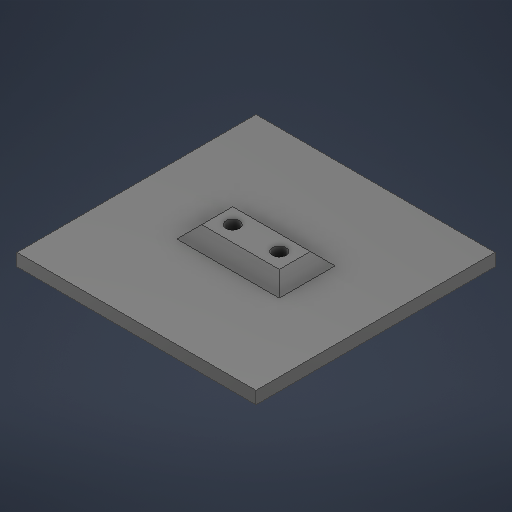
# Autodesk Inventor part: taca
Saved by Autodesk Inventor 2027 (Build 310192060, 192F)
## iProperties
Created: 2026-03-26
Part Number: taca
Material: Ogólny
Document SubType Name: Modeling
Designer: User
Density: 1 g/cm^3
Appearance: Domyślna
Author: User
Autodesk Inventor part; units mm, degrees
ref_plane "YZ Plane" through (0, 0, 0) normal (1, 0, 0) x (0, 1, 0)
ref_plane "XZ Plane" through (0, 0, 0) normal (0, 1, 0) x (-1, 0, 0)
ref_plane "XY Plane" through (0, 0, 0) normal (0, 0, 1) x (1, 0, 0)
sketch "Szkic1" plane through (0, 0, 0) normal (0, 1, 0) x (-1, 0, 0)
  line L0 (0, 0) -> (7.5, 0)
  line L1 (0, 0) -> (7.5, 0) construction
  circle A0 centre (7.5, 0) radius 2.2
  line L2 (0, 0) -> (0, -2)
  circle A1 centre (-7.5, 0) radius 2.2
  line L3 (-38.5, 38.5) -> (38.5, 38.5)
  line L4 (38.5, 38.5) -> (38.5, -38.5)
  line L5 (38.5, -38.5) -> (-38.5, -38.5)
  line L6 (-38.5, -38.5) -> (-38.5, 38.5)
  line L7 (-38.5, 38.5) -> (38.5, -38.5) construction
  line L8 (38.5, 38.5) -> (-38.5, -38.5) construction
  circle A2 centre (7.5, 0) radius 3.5
  circle A3 centre (-7.5, 0) radius 3.5
  dimension "d0" = 7.5
  dimension "d1" = 0
  dimension "d2" = 4.4
  dimension "d3" = 2
  dimension "d4" = 77
  dimension "d5" = 77
  dimension "d8" = 7
  constraints: 18 end point, 4 centre point, 3 horizontal, 2 coincident, 2 midpoint, 2 parallel, 2 symmetric about line, 1 collinear, 1 perpendicular, 1 vertical, 2 other
  measures "d0" distance of L0.start L0.end
  measures "d1" distance between parallel lines of L0 L1
  measures "d2" diameter of A0
  measures "d3" distance of L0.start L2.end
  measures "d4" distance of L4.end L5.end
  measures "d5" distance of L3.end L4.end
  measures "d8" diameter of A2
extrude "Wyciągnięcie proste1" add sketch "Szkic1" along normal blind 6 contours A2 | L3 L4 L5 L6 | A3
extrude "Wyciągnięcie proste2" cut sketch "Szkic1" along normal blind 3 contours A2 | A3
chamfer "Faza1" distance 2 angle 45 4 edges at (-38.5, 0, 0) (0, 0, -38.5) (38.5, 0, 0) (0, 0, 38.5)
sketch "Szkic2" plane through (0, 6, 0) normal (0, 1, 0) x (1, 0, 0)
  line L0 (12.5, -5) -> (-12.5, -5)
  line L1 (-12.5, -5) -> (-12.5, 5)
  line L2 (-12.5, 5) -> (12.5, 5)
  line L3 (12.5, 5) -> (12.5, -5)
  line L4 (12.5, -5) -> (-12.5, 5) construction
  line L5 (-12.5, -5) -> (12.5, 5) construction
  circle A0 centre (-7.5, 0) radius 2.2 projected
  circle A1 centre (-7.5, 0) radius 2.2
  circle A2 centre (7.5, 0) radius 2.2 projected
  circle A3 centre (7.5, 0) radius 2.2
  point P0 (0, 0)
  dimension "d14" = 25
  dimension "d15" = 10
  constraints: 12 end point, 2 centre point, 2 coincident, 2 midpoint, 2 parallel, 1 horizontal, 1 perpendicular
  measures "d14" distance of L1.end L2.end
  measures "d15" distance of L0.end L1.end
extrude "Wyciągnięcie proste3" add sketch "Szkic2" along normal blind 4
chamfer "Faza2" distance 4 angle 45 4 edges at (0, 6, 5) (12.5, 6, 0) (0, 6, -5) (-12.5, 6, 0)
